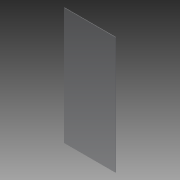
# Autodesk Inventor part: pneumatics board 1
Saved by Autodesk Inventor 2014 (Build 180170000, 170)
## iProperties
Created: 2014-01-20
Part Number: pneumatics board 1
Material: Polycarbonate, Clear
Document SubType Name: Modeling
Designer: Arpan
Density: 1.2 g/cm^3
Appearance: Polycarbonate - Clear
Author: Arpan
Autodesk Inventor part; units mm, degrees
ref_plane "YZ Plane" through (0, 0, 0) normal (1, 0, 0) x (0, 1, 0)
ref_plane "XZ Plane" through (0, 0, 0) normal (0, 1, 0) x (-1, 0, 0)
ref_plane "XY Plane" through (0, 0, 0) normal (0, 0, 1) x (1, 0, 0)
sketch "Sketch1" plane through (0, 0, 0) normal (0, 0, 1) x (1, 0, 0)
  line L0 (0, 0) -> (-150.114, 0)
  line L1 (-150.114, 0) -> (-150.114, 418.8714)
  line L2 (-150.114, 418.8714) -> (0, 418.8714)
  line L3 (0, 418.8714) -> (0, 0)
  dimension "d0" = 150.114
  dimension "d1" = 418.8714
  constraints: 8 end point, 2 parallel, 1 horizontal, 1 perpendicular
  measures "d0" distance of L1.end L2.end
  measures "d1" distance of L2.end L0.start
extrude "Extrusion1" add sketch "Sketch1" along normal blind 1.5875
body "Solid1"
